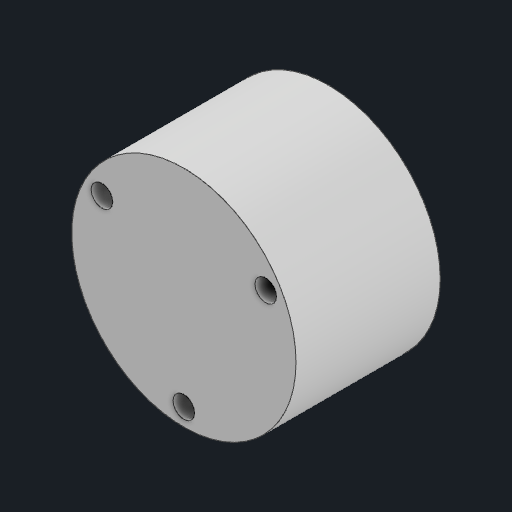
# Autodesk Inventor part: Hoverboard Frame
Saved by Autodesk Inventor 2022.2 (Build 262287000, 287)
## iProperties
Created: 2022-11-11
Part Number: Hoverboard Frame
Material: Generic
Document SubType Name: Modeling
Designer: haash
Density: 1 g/cm^3
Appearance: Default
Author: haash
Autodesk Inventor part; units mm, degrees
ref_plane "YZ Plane" through (0, 0, 0) normal (1, 0, 0) x (0, 1, 0)
ref_plane "XZ Plane" through (0, 0, 0) normal (0, 1, 0) x (-1, 0, 0)
ref_plane "XY Plane" through (0, 0, 0) normal (0, 0, 1) x (1, 0, 0)
sketch "Sketch1" plane through (0, 0, 0) normal (0, 0, 1) x (1, 0, 0)
  circle A0 centre (0, 0) radius 20.75
  dimension "d0" = 41.5
  constraints: 1 centre point, 1 coincident
  measures "d0" diameter of A0
extrude "Extrusion1" add sketch "Sketch1" along normal blind 26.7
sketch "Sketch2" plane through (0, 0, 26.7) normal (0, 0, 1) x (1, 0, 0)
  circle A0 centre (-15.1554, 8.75) radius 2
  circle A1 centre (15.1554, 8.75) radius 2
  circle A2 centre (0, -17.5) radius 2
  circle A3 centre (0, 0) radius 17.5 construction
  line L0 (0, 0) -> (-15.1554, 8.75) construction
  line L1 (0, 0) -> (15.1554, 8.75) construction
  line L2 (0, 0) -> (0, -17.5) construction
  dimension "d3" = 35
  dimension "d4" = 120
  dimension "d5" = 120
  dimension "d6" = 4
  constraints: 6 end point, 4 centre point, 3 point on circle, 2 equal radius, 1 coincident, 1 vertical
  measures "d3" diameter of A3
  measures "d4" angle of L0 L2
  measures "d5" angle of L1 L0
  measures "d6" diameter of A1
extrude "Extrusion2" cut sketch "Sketch2" against normal blind 20
body "Solid1"
